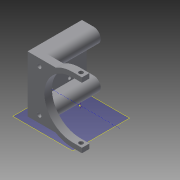
# Autodesk Inventor part: base
Saved by Autodesk Inventor 2015 SP2 (Build 190223200, 223)
## iProperties
Created: 2016-03-05
Part Number: base
Material: Generic
Document SubType Name: Modeling
Designer: marc
Density: 1 g/cm^3
Appearance: Default
Author: marc
Autodesk Inventor part; units mm, degrees
ref_plane "YZ Plane" through (0, 0, 0) normal (1, 0, 0) x (0, 1, 0)
ref_plane "XZ Plane" through (0, 0, 0) normal (0, 1, 0) x (-1, 0, 0)
ref_plane "XY Plane" through (0, 0, 0) normal (0, 0, 1) x (1, 0, 0)
sketch "Sketch1" plane through (0, 0, 0) normal (0, 1, 0) x (-1, 0, 0)
  arc A0 (0, -30) -> (0, 30) centre (0, 0) ccw
  arc A1 (0, -35) -> (0, 35) centre (0, 0) ccw
  line L0 (0, 66.4807) -> (0, -80.0863) construction
  line L1 (-55.1659, 0) -> (60.8047, 0) construction
  line L2 (18.0278, 30) -> (48.0278, 30)
  line L3 (48.0278, 30) -> (48.0278, -30)
  line L4 (48.0278, -30) -> (18.0278, -30)
  line L5 (18.0278, 30) -> (48.0278, -30) construction
  line L6 (48.0278, 30) -> (18.0278, -30) construction
  line L7 (18.0278, 30) -> (18.0278, -30) construction
  line L8 (0, 35) -> (-10, 35)
  line L9 (0, 30) -> (-10, 30)
  line L10 (-10, 35) -> (-10, 30)
  line L11 (0, -35) -> (-10, -35)
  line L12 (0, -30) -> (-10, -30)
  line L13 (-10, -35) -> (-10, -30)
  point P0 (33.0278, 0)
  dimension "diameterCylinder" = 60
  dimension "thicknessFlange" = 5
  dimension "widthC" = 60
  dimension "offsetC" = 30
  dimension "d33" = 10
  constraints: 28 end point, 7 point on line, 6 point on circle, 4 horizontal, 2 centre point, 2 coincident, 2 midpoint, 2 parallel, 2 symmetric about line, 2 vertical, 1 perpendicular
  measures "diameterCylinder" diameter of A0
  measures "thicknessFlange" radial gap between concentric circles of A1 A0
  measures "widthC" distance of L2.end L3.end
  measures "offsetC" distance from line of L4.end L3
  measures "d33" distance between parallel lines of L0 L10
extrude "Extrusion1" add sketch "Sketch1" along normal blind 8
sketch "Sketch2" plane through (0, 8, 0) normal (0, 1, 0) x (1, 0, 0)
  line L0 (-18.0278, 30) -> (-48.0278, 30) projected
  line L1 (-48.0278, -30) -> (-43.0278, -30)
  line L2 (-43.0278, -30) -> (-43.0278, 30)
  line L3 (-43.0278, 30) -> (-48.0278, 30)
  line L4 (-48.0278, 30) -> (-48.0278, -30)
  point P0 (0, 0)
  dimension "thicknessC" = 5
  constraints: 8 end point, 2 parallel, 1 horizontal, 1 perpendicular, 1 point on line
  measures "thicknessC" distance between parallel lines of L4 L2
extrude "Extrusion2" add sketch "Sketch2" along normal blind 50
sketch "Sketch3" plane through (0, 8, 0) normal (0, 1, 0) x (1, 0, 0)
  circle A0 centre (-35.5278, -22.5) radius 7.5
  line L0 (-35.5278, -30) -> (-48.0278, -30)
  line L1 (-48.0278, 30) -> (-48.0278, -30) projected
  line L2 (-48.0278, -30) -> (-48.0278, -15)
  line L3 (-48.0278, -15) -> (-35.5278, -15)
  line L4 (0, 0) -> (-116.9201, 0) construction
  line L5 (-43.0278, -30) -> (-43.0278, 30) construction
  line L6 (-43.0278, -30) -> (-18.0278, -30) construction
  circle A1 centre (-35.5278, 22.5) radius 7.5
  line L7 (-35.5278, 30) -> (-48.0278, 30)
  line L8 (-48.0278, -30) -> (-48.0278, 30)
  line L9 (-48.0278, 15) -> (-35.5278, 15)
  dimension "d35" = 15
  constraints: 14 end point, 7 symmetric about line, 4 point on circle, 4 point on line, 3 tangent, 2 centre point, 2 horizontal, 1 collinear, 1 parallel, 1 other
  measures "d35" diameter of A0
extrude "Extrusion3" add sketch "Sketch3" along normal up to surface (50 mm away)
sketch "Sketch4" plane through (-48.0278, 0, -30) normal (-1, 0, 0) x (0, 0, 1)
  line L0 (30, 0) -> (30, 84.984) construction
  line L1 (18, 20) -> (42, 20) construction
  line L2 (42, 20) -> (42, 40) construction
  line L3 (42, 40) -> (18, 40) construction
  line L4 (18, 40) -> (18, 20) construction
  line L5 (18, 20) -> (42, 40) construction
  line L6 (42, 20) -> (18, 40) construction
  line L7 (0, 0) -> (60, 0) construction
  point P0 (30, 30)
  dimension "holespacingZ" = 24
  dimension "holeSpacingY" = 20
  dimension "holeOffset" = 30
  constraints: 14 end point, 4 coincident, 2 midpoint, 2 parallel, 1 horizontal, 1 perpendicular, 1 point on line, 1 vertical
  measures "holespacingZ" distance of L2.end L3.end
  measures "holeSpacingY" distance between parallel lines of L1 L3
  measures "holeOffset" distance from line of L7 point (30, 30)
hole "Hole1" at (-48.0278, 40, -12) at (-48.0278, 40, 12) at (-48.0278, 20, 12) at (-48.0278, 20, -12) direction (1, 0, 0) diameter 3.4 end through all clearance for "Socket Head Cap Screw ISO 4762" size "M3" standard "ISO"
ref_plane "Work Plane1" through (0, 0, -35) normal (0, 0, -1) x (-1, 0, 0)
sketch "Sketch5" plane through (0, 0, -35) normal (0, 0, -1) x (-1, 0, 0)
  line L0 (0, 0) -> (0, 8) projected
  line L1 (-10, 0) -> (-10, 8) projected
  point P0 (-5, 4)
  dimension "holePosistionYF" = 4
  dimension "d34" = 5
  measures "holePosistionYF" vertical distance of L0.start point (-5, 4)
  measures "d34" distance from line of L1 point (-5, 4)
hole "Hole2" at (5, 4, -35) direction (0, 0, 1) diameter 4.5 end through all clearance for "Socket Head Cap Screw ISO 4762" size "M4" standard "ISO"
sketch "Sketch7" plane through (0, 8, 0) normal (0, 1, 0) x (1, 0, 0)
  line L0 (-50.9329, 0) -> (42.7836, 0) construction
  point P0 (0, 0)
  point P1 (0, 0)
  constraints: 2 end point, 1 coincident, 1 horizontal, 1 point on line
sketch "Sketch8" plane through (0, 58, 0) normal (0, 1, 0) x (1, 0, 0)
  circle A0 centre (-35.5278, -22.5) radius 4.3737 construction
  arc A1 (-35.5278, -30) -> (-35.5278, -15) centre (-35.5278, -22.5) ccw construction
  line L0 (0, 0) -> (-70.9359, 0) construction
  circle A2 centre (-35.5278, 22.5) radius 4.3737 construction
  constraints: 2 centre point, 2 coincident, 2 end point, 1 concentric, 1 horizontal, 1 symmetric about line, 1 other
hole "Hole3" at (-35.5278, 58, 22.5) at (-35.5278, 58, -22.5) direction (0, -1, 0) diameter 4.5 end through all clearance for "Hex Head Machine Screw" size "M4" standard "Ansi Metric M Profile"
sketch "Sketch9" plane through (0, 58, 0) normal (0, 1, 0) x (1, 0, 0)
  circle A0 centre (-35.5278, -22.5) radius 5.085 construction
  arc A1 (-35.5278, -30) -> (-35.5278, -15) centre (-35.5278, -22.5) ccw construction
  line L0 (-39.4928, -20.2108) -> (-35.5278, -17.9216)
  line L1 (-35.5278, -17.9216) -> (-31.5628, -20.2108)
  line L2 (-31.5628, -20.2108) -> (-31.5628, -24.7892)
  line L3 (-31.5628, -24.7892) -> (-35.5278, -27.0784)
  line L4 (-35.5278, -27.0784) -> (-39.4928, -24.7892)
  line L5 (-39.4928, -24.7892) -> (-39.4928, -20.2108)
  line L6 (-48.0278, 30) -> (-48.0278, -30) projected
  line L7 (0, 0) -> (-58.3067, 0) construction
  line L8 (-39.4928, 20.2108) -> (-35.5278, 17.9216)
  line L9 (-35.5278, 17.9216) -> (-31.5628, 20.2108)
  line L10 (-31.5628, 20.2108) -> (-31.5628, 24.7892)
  line L11 (-31.5628, 24.7892) -> (-35.5278, 27.0784)
  line L12 (-35.5278, 27.0784) -> (-39.4928, 24.7892)
  line L13 (-39.4928, 24.7892) -> (-39.4928, 20.2108)
  dimension "nutSlotHeight" = 7.93
  constraints: 26 end point, 6 symmetric about line, 1 centre point, 1 coincident, 1 concentric, 1 horizontal, 1 parallel, 13 other
  measures "nutSlotHeight" distance between parallel lines of L2 L5
extrude "Extrusion4" cut sketch "Sketch9" against normal blind 4
equation "\"holePosistionYF\" = 0.5 * flangeHeigth"
equation "\"flangeHeigth\" = 8"
body "Solid1"
